Autodesk Fusion 360 part; units mm, degrees
(part 2 of 2)
sketch "Sketch2 (2)" plane through (0, 0, 0) normal (-1, 0, 0) x (0, -1, 0) in component "left"
  line L0 (-22.5, 130) -> (-22.5, 127)
  line L1 (-22.5, 127) -> (-32.1429, 127)
  line L2 (-32.1429, 127) -> (-32.1429, 130)
  line L3 (-32.1429, 130) -> (-42.8571, 130)
  line L4 (-42.8571, 130) -> (-42.8571, 127)
  line L5 (-42.8571, 127) -> (-52.5, 127)
  line L6 (-52.5, 127) -> (-52.5, 130)
  line L7 (-52.5, 130) -> (-52.5, 200)
  line L8 (-52.5, 200) -> (-72, 200)
  line L9 (-72, 200) -> (-72, 177.7778)
  line L10 (-72, 177.7778) -> (-75, 177.7778)
  line L11 (-75, 177.7778) -> (-75, 155.5556)
  line L12 (-75, 155.5556) -> (-72, 155.5556)
  line L13 (-72, 155.5556) -> (-72, 133.3333)
  line L14 (-72, 133.3333) -> (-75, 133.3333)
  line L15 (-75, 133.3333) -> (-75, 111.1111)
  line L16 (-75, 111.1111) -> (-72, 111.1111)
  line L17 (-72, 111.1111) -> (-72, 88.8889)
  line L18 (-72, 88.8889) -> (-75, 88.8889)
  line L19 (-75, 88.8889) -> (-75, 66.6667)
  line L20 (-75, 66.6667) -> (-72, 66.6667)
  line L21 (-72, 66.6667) -> (-72, 44.4444)
  line L22 (-72, 44.4444) -> (-75, 44.4444)
  line L23 (-75, 44.4444) -> (-75, 22.2222)
  line L24 (-75, 22.2222) -> (-72, 22.2222)
  line L25 (-72, 22.2222) -> (-72, 3)
  line L26 (-72, 3) -> (-64.2857, 3)
  line L27 (-64.2857, 3) -> (-64.2857, 0)
  line L28 (-64.2857, 0) -> (-53.5714, 0)
  line L29 (-53.5714, 0) -> (-53.5714, 3)
  line L30 (-53.5714, 3) -> (-42.8571, 3)
  line L31 (-42.8571, 3) -> (-42.8571, 0)
  line L32 (-42.8571, 0) -> (-32.1429, 0)
  line L33 (-32.1429, 0) -> (-32.1429, 3)
  line L34 (-32.1429, 3) -> (-21.4286, 3)
  line L35 (-21.4286, 3) -> (-21.4286, 0)
  line L36 (-21.4286, 0) -> (-10.7143, 0)
  line L37 (-10.7143, 0) -> (-10.7143, 3)
  line L38 (-10.7143, 3) -> (-3, 3)
  line L39 (-3, 3) -> (-3, 22.2222)
  line L40 (-3, 22.2222) -> (0, 22.2222)
  line L41 (0, 22.2222) -> (0, 44.4444)
  line L42 (0, 44.4444) -> (-3, 44.4444)
  line L43 (-3, 44.4444) -> (-3, 66.6667)
  line L44 (-3, 66.6667) -> (0, 66.6667)
  line L45 (0, 66.6667) -> (0, 88.8889)
  line L46 (0, 88.8889) -> (-3, 88.8889)
  line L47 (-3, 88.8889) -> (-3, 111.1111)
  line L48 (-3, 111.1111) -> (0, 111.1111)
  line L49 (0, 111.1111) -> (0, 133.3333)
  line L50 (0, 133.3333) -> (-3, 133.3333)
  line L51 (-3, 133.3333) -> (-3, 155.5556)
  line L52 (-3, 155.5556) -> (0, 155.5556)
  line L53 (0, 155.5556) -> (0, 177.7778)
  line L54 (0, 177.7778) -> (-3, 177.7778)
  line L55 (-3, 177.7778) -> (-3, 200)
  line L56 (-3, 200) -> (-22.5, 200)
  line L57 (-22.5, 200) -> (-22.5, 130)
  line L58 (-52.5, 200) -> (-22.5, 200)
  line L59 (-22.5, 200) -> (-22.5, 156)
  line L60 (-22.5, 156) -> (-52.5, 156)
  line L61 (-52.5, 156) -> (-52.5, 200)
  dimension "d161" = 26
  constraint horizontal L58
  constraint vertical L59
  constraint horizontal L60
  constraint vertical L61
  constraint coincident L57 L59.end
  constraint coincident L7.end L8.start
  measures "d161" distance of L3 L60
extrude "Extrude4'''" add sketch "Sketch2 (2)" against normal blind 3 contours L7 L57 L58 L59 L60 L61 bodies 5 in component "left"
combine "Combine6" operation cut target body 4 tool bodies 8 keep tools in component "right"
sketch "Sketch3 (2)" plane through (0, 0, 0) normal (-1, 0, 0) x (0, -1, 0) in component "left"
  line L0 (-22.5, 156) -> (-22.5, 130)
  line L1 (-22.5, 130) -> (-22.5, 127)
  line L2 (-22.5, 127) -> (-32.1429, 127)
  line L3 (-32.1429, 127) -> (-32.1429, 130)
  line L4 (-32.1429, 130) -> (-42.8571, 130)
  line L5 (-42.8571, 130) -> (-42.8571, 127)
  line L6 (-42.8571, 127) -> (-52.5, 127)
  line L7 (-52.5, 127) -> (-52.5, 130)
  line L8 (-52.5, 130) -> (-52.5, 156)
  line L9 (-52.5, 156) -> (-22.5, 156)
  line L10 (-3, 200) -> (-72, 200)
  line L11 (-72, 200) -> (-72, 177.7778)
  line L12 (-72, 177.7778) -> (-75, 177.7778)
  line L13 (-75, 177.7778) -> (-75, 155.5556)
  line L14 (-75, 155.5556) -> (-72, 155.5556)
  line L15 (-72, 155.5556) -> (-72, 133.3333)
  line L16 (-72, 133.3333) -> (-75, 133.3333)
  line L17 (-75, 133.3333) -> (-75, 111.1111)
  line L18 (-75, 111.1111) -> (-72, 111.1111)
  line L19 (-72, 111.1111) -> (-72, 88.8889)
  line L20 (-72, 88.8889) -> (-75, 88.8889)
  line L21 (-75, 88.8889) -> (-75, 66.6667)
  line L22 (-75, 66.6667) -> (-72, 66.6667)
  line L23 (-72, 66.6667) -> (-72, 44.4444)
  line L24 (-72, 44.4444) -> (-75, 44.4444)
  line L25 (-75, 44.4444) -> (-75, 22.2222)
  line L26 (-75, 22.2222) -> (-72, 22.2222)
  line L27 (-72, 22.2222) -> (-72, 3)
  line L28 (-72, 3) -> (-64.2857, 3)
  line L29 (-64.2857, 3) -> (-64.2857, 0)
  line L30 (-64.2857, 0) -> (-53.5714, 0)
  line L31 (-53.5714, 0) -> (-53.5714, 3)
  line L32 (-53.5714, 3) -> (-42.8571, 3)
  line L33 (-42.8571, 3) -> (-42.8571, 0)
  line L34 (-42.8571, 0) -> (-32.1429, 0)
  line L35 (-32.1429, 0) -> (-32.1429, 3)
  line L36 (-32.1429, 3) -> (-21.4286, 3)
  line L37 (-21.4286, 3) -> (-21.4286, 0)
  line L38 (-21.4286, 0) -> (-10.7143, 0)
  line L39 (-10.7143, 0) -> (-10.7143, 3)
  line L40 (-10.7143, 3) -> (-3, 3)
  line L41 (-3, 3) -> (-3, 22.2222)
  line L42 (-3, 22.2222) -> (0, 22.2222)
  line L43 (0, 22.2222) -> (0, 44.4444)
  line L44 (0, 44.4444) -> (-3, 44.4444)
  line L45 (-3, 44.4444) -> (-3, 66.6667)
  line L46 (-3, 66.6667) -> (0, 66.6667)
  line L47 (0, 66.6667) -> (0, 88.8889)
  line L48 (0, 88.8889) -> (-3, 88.8889)
  line L49 (-3, 88.8889) -> (-3, 111.1111)
  line L50 (-3, 111.1111) -> (0, 111.1111)
  line L51 (0, 111.1111) -> (0, 133.3333)
  line L52 (0, 133.3333) -> (-3, 133.3333)
  line L53 (-3, 133.3333) -> (-3, 155.5556)
  line L54 (-3, 155.5556) -> (0, 155.5556)
  line L55 (0, 155.5556) -> (0, 177.7778)
  line L56 (0, 177.7778) -> (-3, 177.7778)
  line L57 (-3, 177.7778) -> (-3, 200)
  circle A0 centre (-60, 117) radius 2.5
  dimension "d164" = 10
  dimension "d165" = 5
  dimension "d166" = 15
  measures "d164" distance of L6 A0.centre
  measures "d165" diameter of A0
  measures "d166" distance of L17 A0.centre
extrude "Extrude5'''" cut sketch "Sketch3 (2)" against normal blind 3 contours A0 bodies 5 in component "left"
sketch "Sketch7" plane through (75, 0, 0) normal (1, 0, 0) x (0, 1, 0) in component "right"
  line L0 (72, 78) -> (72, 66.6667)
  line L1 (72, 66.6667) -> (75, 66.6667)
  line L2 (75, 66.6667) -> (75, 88.8889)
  line L3 (75, 88.8889) -> (72, 88.8889)
  line L4 (72, 88.8889) -> (72, 111.1111)
  line L5 (72, 111.1111) -> (75, 111.1111)
  line L6 (75, 111.1111) -> (75, 133.3333)
  line L7 (75, 133.3333) -> (72, 133.3333)
  line L8 (72, 133.3333) -> (72, 155.5556)
  line L9 (72, 155.5556) -> (75, 155.5556)
  line L10 (75, 155.5556) -> (75, 177.7778)
  line L11 (75, 177.7778) -> (72, 177.7778)
  line L12 (72, 177.7778) -> (72, 200)
  line L13 (72, 200) -> (3, 200)
  line L14 (3, 200) -> (3, 177.7778)
  line L15 (3, 177.7778) -> (0, 177.7778)
  line L16 (0, 177.7778) -> (0, 155.5556)
  line L17 (0, 155.5556) -> (3, 155.5556)
  line L18 (3, 155.5556) -> (3, 133.3333)
  line L19 (3, 133.3333) -> (0, 133.3333)
  line L20 (0, 133.3333) -> (0, 111.1111)
  line L21 (0, 111.1111) -> (3, 111.1111)
  line L22 (3, 111.1111) -> (3, 88.8889)
  line L23 (3, 88.8889) -> (0, 88.8889)
  line L24 (0, 88.8889) -> (0, 66.6667)
  line L25 (0, 66.6667) -> (3, 66.6667)
  line L26 (3, 66.6667) -> (3, 44.4444)
  line L27 (3, 44.4444) -> (0, 44.4444)
  line L28 (0, 44.4444) -> (0, 22.2222)
  line L29 (0, 22.2222) -> (3, 22.2222)
  line L30 (3, 22.2222) -> (3, 3)
  line L31 (3, 3) -> (10.7143, 3)
  line L32 (10.7143, 3) -> (10.7143, 0)
  line L33 (10.7143, 0) -> (21.4286, 0)
  line L34 (21.4286, 0) -> (21.4286, 3)
  line L35 (21.4286, 3) -> (32.1429, 3)
  line L36 (32.1429, 3) -> (32.1429, 0)
  line L37 (32.1429, 0) -> (42.8571, 0)
  line L38 (42.8571, 0) -> (42.8571, 3)
  line L39 (42.8571, 3) -> (53.5714, 3)
  line L40 (53.5714, 3) -> (53.5714, 0)
  line L41 (53.5714, 0) -> (64.2857, 0)
  line L42 (64.2857, 0) -> (64.2857, 3)
  line L43 (64.2857, 3) -> (69, 3)
  line L44 (69, 3) -> (69, 78)
  line L45 (69, 78) -> (72, 78)
  circle A0 centre (60, 117) radius 2.5
  line L46 (52.5, 127) -> (42.8571, 127)
  line L47 (75, 0) -> (75, 200)
  dimension "d171" = 5
  dimension "d190" = 10
  dimension "d191" = 15
  measures "d171" diameter of A0
  measures "d190" distance of A0.centre L46
  measures "d191" distance of A0.centre L47
extrude "Extrude8" cut sketch "Sketch7" against normal blind 8 contours A0 bodies 4 in component "right"
sketch "Sketch3 (3)" plane through (0, 0, 0) normal (0, -1, 0) x (1, 0, 0) in component "front"
  line L0 (52.5, 156) -> (52.5, 130)
  line L1 (52.5, 130) -> (50, 130)
  line L2 (50, 130) -> (50, 127)
  line L3 (50, 127) -> (41.6667, 127)
  line L4 (41.6667, 127) -> (41.6667, 130)
  line L5 (41.6667, 130) -> (33.3333, 130)
  line L6 (33.3333, 130) -> (33.3333, 127)
  line L7 (33.3333, 127) -> (25, 127)
  line L8 (25, 127) -> (25, 130)
  line L9 (25, 130) -> (22.5, 130)
  line L10 (22.5, 130) -> (22.5, 156)
  line L11 (22.5, 156) -> (52.5, 156)
  line L12 (75, 200) -> (0, 200)
  line L13 (0, 200) -> (0, 177.7778)
  line L14 (0, 177.7778) -> (3, 177.7778)
  line L15 (3, 177.7778) -> (3, 155.5556)
  line L16 (3, 155.5556) -> (0, 155.5556)
  line L17 (0, 155.5556) -> (0, 133.3333)
  line L18 (0, 133.3333) -> (3, 133.3333)
  line L19 (3, 133.3333) -> (3, 111.1111)
  line L20 (3, 111.1111) -> (0, 111.1111)
  line L21 (0, 111.1111) -> (0, 88.8889)
  line L22 (0, 88.8889) -> (3, 88.8889)
  line L23 (3, 88.8889) -> (3, 66.6667)
  line L24 (3, 66.6667) -> (0, 66.6667)
  line L25 (0, 66.6667) -> (0, 44.4444)
  line L26 (0, 44.4444) -> (3, 44.4444)
  line L27 (3, 44.4444) -> (3, 22.2222)
  line L28 (3, 22.2222) -> (0, 22.2222)
  line L29 (0, 22.2222) -> (0, 3)
  line L30 (0, 3) -> (8.3333, 3)
  line L31 (8.3333, 3) -> (8.3333, 0)
  line L32 (8.3333, 0) -> (16.6667, 0)
  line L33 (16.6667, 0) -> (16.6667, 3)
  line L34 (16.6667, 3) -> (25, 3)
  line L35 (25, 3) -> (25, 0)
  line L36 (25, 0) -> (33.3333, 0)
  line L37 (33.3333, 0) -> (33.3333, 3)
  line L38 (33.3333, 3) -> (41.6667, 3)
  line L39 (41.6667, 3) -> (41.6667, 0)
  line L40 (41.6667, 0) -> (50, 0)
  line L41 (50, 0) -> (50, 3)
  line L42 (50, 3) -> (58.3333, 3)
  line L43 (58.3333, 3) -> (58.3333, 0)
  line L44 (58.3333, 0) -> (66.6667, 0)
  line L45 (66.6667, 0) -> (66.6667, 3)
  line L46 (66.6667, 3) -> (75, 3)
  line L47 (75, 3) -> (75, 22.2222)
  line L48 (75, 22.2222) -> (72, 22.2222)
  line L49 (72, 22.2222) -> (72, 44.4444)
  line L50 (72, 44.4444) -> (75, 44.4444)
  line L51 (75, 44.4444) -> (75, 66.6667)
  line L52 (75, 66.6667) -> (72, 66.6667)
  line L53 (72, 66.6667) -> (72, 88.8889)
  line L54 (72, 88.8889) -> (75, 88.8889)
  line L55 (75, 88.8889) -> (75, 111.1111)
  line L56 (75, 111.1111) -> (72, 111.1111)
  line L57 (72, 111.1111) -> (72, 133.3333)
  line L58 (72, 133.3333) -> (75, 133.3333)
  line L59 (75, 133.3333) -> (75, 155.5556)
  line L60 (75, 155.5556) -> (72, 155.5556)
  line L61 (72, 155.5556) -> (72, 177.7778)
  line L62 (72, 177.7778) -> (75, 177.7778)
  line L63 (75, 177.7778) -> (75, 200)
  circle A0 centre (18, 117) radius 2.5
  dimension "d174" = 10
  dimension "d175" = 15
  dimension "d176" = 5
  measures "d174" distance of L7 A0.centre
  measures "d175" distance of L19 A0.centre
  measures "d176" diameter of A0
extrude "Extrude5''''" cut sketch "Sketch3 (3)" against normal blind 3 contours A0 bodies 3 in component "front"
sketch "Sketch6 (2)" plane through (0, 72, 0) normal (0, -1, 0) x (1, 0, 0) in component "back"
  line L0 (13, 8) -> (13, 78)
  line L1 (13, 78) -> (62, 78)
  line L2 (62, 78) -> (62, 8)
  line L3 (62, 8) -> (13, 8)
  line L4 (0, 3) -> (8.3333, 3)
  line L5 (8.3333, 3) -> (8.3333, 0)
  line L6 (8.3333, 0) -> (16.6667, 0)
  line L7 (16.6667, 0) -> (16.6667, 3)
  line L8 (16.6667, 3) -> (25, 3)
  line L9 (25, 3) -> (25, 0)
  line L10 (25, 0) -> (33.3333, 0)
  line L11 (33.3333, 0) -> (33.3333, 3)
  line L12 (33.3333, 3) -> (41.6667, 3)
  line L13 (41.6667, 3) -> (41.6667, 0)
  line L14 (41.6667, 0) -> (50, 0)
  line L15 (50, 0) -> (50, 3)
  line L16 (50, 3) -> (58.3333, 3)
  line L17 (58.3333, 3) -> (58.3333, 0)
  line L18 (58.3333, 0) -> (66.6667, 0)
  line L19 (66.6667, 0) -> (66.6667, 3)
  line L20 (66.6667, 3) -> (75, 3)
  line L21 (75, 3) -> (75, 22.2222)
  line L22 (75, 22.2222) -> (75, 44.4444)
  line L23 (75, 44.4444) -> (75, 66.6667)
  line L24 (75, 66.6667) -> (72, 66.6667)
  line L25 (72, 66.6667) -> (72, 88.8889)
  line L26 (72, 88.8889) -> (75, 88.8889)
  line L27 (75, 88.8889) -> (75, 111.1111)
  line L28 (75, 111.1111) -> (72, 111.1111)
  line L29 (72, 111.1111) -> (72, 133.3333)
  line L30 (72, 133.3333) -> (75, 133.3333)
  line L31 (75, 133.3333) -> (75, 155.5556)
  line L32 (75, 155.5556) -> (72, 155.5556)
  line L33 (72, 155.5556) -> (72, 177.7778)
  line L34 (72, 177.7778) -> (75, 177.7778)
  line L35 (75, 177.7778) -> (75, 200)
  line L36 (75, 200) -> (0, 200)
  line L37 (0, 200) -> (0, 177.7778)
  line L38 (0, 177.7778) -> (3, 177.7778)
  line L39 (3, 177.7778) -> (3, 155.5556)
  line L40 (3, 155.5556) -> (0, 155.5556)
  line L41 (0, 155.5556) -> (0, 133.3333)
  line L42 (0, 133.3333) -> (3, 133.3333)
  line L43 (3, 133.3333) -> (3, 111.1111)
  line L44 (3, 111.1111) -> (0, 111.1111)
  line L45 (0, 111.1111) -> (0, 88.8889)
  line L46 (0, 88.8889) -> (3, 88.8889)
  line L47 (3, 88.8889) -> (3, 66.6667)
  line L48 (3, 66.6667) -> (0, 66.6667)
  line L49 (0, 66.6667) -> (0, 44.4444)
  line L50 (0, 44.4444) -> (3, 44.4444)
  line L51 (3, 44.4444) -> (3, 22.2222)
  line L52 (3, 22.2222) -> (0, 22.2222)
  line L53 (0, 22.2222) -> (0, 3)
  circle A0 centre (37.5, 117) radius 2.5
  line L54 (3, 127) -> (72, 127)
  line L55 (37.5, 117) -> (37.5, 127)
  dimension "d183" = 5
  dimension "d186" = 10
  constraint coincident A0.centre L55.start
  constraint coincident L54 L55.end
  constraint perpendicular L54 L55
  constraint midpoint L54 L55.end
  measures "d183" diameter of A0
  measures "d186" distance of A0.centre L55.end
extrude "Extrude7'" cut sketch "Sketch6 (2)" against normal blind 6 contours A0 bodies 2 in component "back"
extrude "Extrude9" cut sketch "spout_cut" against normal blind 10 contours L30 L48 L49 L50 L51 bodies 4 in component "right"
sketch "Sketch8" plane through (75, 0, 0) normal (1, 0, 0) x (0, 1, 0) in component "right"
  line L0 (52.5, 156) -> (22.5, 156)
  line L1 (22.5, 156) -> (22.5, 200)
  line L2 (22.5, 200) -> (52.5, 200)
  line L3 (52.5, 200) -> (52.5, 156)
  line L4 (22.5, 156) -> (52.5, 156)
  line L5 (52.5, 200) -> (52.5, 130)
  point P0 (22.5, 200)
  constraint horizontal L0
  constraint vertical L1
  constraint horizontal L2
  constraint vertical L3
  constraint coincident P0 L1.end
  constraint coincident L0.start L4
  constraint coincident L2.end L5
extrude "Extrude10" add sketch "Sketch8" against normal blind 3 bodies 4 in component "right"
combine "Combine7" operation cut target body 4 tool bodies 6 keep tools in component "right"
sketch "Sketch1 (5)" plane through (0, 0, 200) normal (0, 0, 1) x (-1, 0, 0) in component "cover"
  line L0 (-75, -75) -> (0, -75)
  line L1 (0, -75) -> (0, -72)
  line L2 (0, -72) -> (-75, -72)
  line L3 (-75, -72) -> (-75, -75)
  line L4 (-75, -75) -> (0, -75)
  line L5 (0, -75) -> (0, 0)
  line L6 (0, 0) -> (-75, 0)
  line L7 (-75, 0) -> (-75, -75)
  line L8 (5, 5) -> (-80, 5)
  line L9 (-80, 5) -> (-80, -80)
  line L10 (-80, -80) -> (5, -80)
  line L11 (5, -80) -> (5, 5)
  line L12 (0, -64.2857) -> (-3, -64.2857)
  line L13 (-3, -64.2857) -> (-3, -53.5714)
  line L14 (-3, -53.5714) -> (0, -53.5714)
  line L15 (0, -53.5714) -> (0, -64.2857)
  line L16 (0, -64.2857) -> (-3, -64.2857)
  line L17 (-3, -53.5714) -> (0, -53.5714)
  line L18 (-3, -42.8571) -> (0, -42.8571)
  line L19 (0, -42.8571) -> (0, -32.1429)
  line L20 (0, -32.1429) -> (-3, -32.1429)
  line L21 (-3, -32.1429) -> (-3, -42.8571)
  line L22 (-3, -21.4286) -> (0, -21.4286)
  line L23 (0, -21.4286) -> (0, -10.7143)
  line L24 (0, -10.7143) -> (-3, -10.7143)
  line L25 (-3, -10.7143) -> (-3, -21.4286)
  line L26 (0, -21.4286) -> (-3, -21.4286)
  line L27 (-3, -32.1429) -> (0, -32.1429)
  line L28 (-16.6667, -75) -> (-8.3333, -75)
  line L29 (-8.3333, -75) -> (-8.3333, -72)
  line L30 (-8.3333, -72) -> (-16.6667, -72)
  line L31 (-16.6667, -72) -> (-16.6667, -75)
  line L32 (-33.3333, -75) -> (-25, -75)
  line L33 (-25, -75) -> (-25, -72)
  line L34 (-25, -72) -> (-33.3333, -72)
  line L35 (-33.3333, -72) -> (-33.3333, -75)
  line L36 (-50, -75) -> (-41.6667, -75)
  line L37 (-41.6667, -75) -> (-41.6667, -72)
  line L38 (-41.6667, -72) -> (-50, -72)
  line L39 (-50, -72) -> (-50, -75)
  line L40 (-66.6667, -75) -> (-58.3333, -75)
  line L41 (-58.3333, -75) -> (-58.3333, -72)
  line L42 (-58.3333, -72) -> (-66.6667, -72)
  line L43 (-66.6667, -72) -> (-66.6667, -75)
  line L44 (-8.3333, -72) -> (-8.3333, -75)
  line L45 (-16.6667, -75) -> (-16.6667, -72)
  line L46 (-25, -72) -> (-25, -75)
  line L47 (-33.3333, -75) -> (-33.3333, -72)
  line L48 (-41.6667, -72) -> (-41.6667, -75)
  line L49 (-58.3333, -72) -> (-58.3333, -75)
  line L50 (-66.6667, -75) -> (-66.6667, -72)
  line L51 (5, -37.5) -> (-80, -37.5) construction
  line L52 (-37.5, -80) -> (-37.5, 5) construction
  line L53 (-72, -42.8571) -> (-75, -42.8571)
  line L54 (-75, -21.4286) -> (-75, -10.7143)
  line L55 (-72, -64.2857) -> (-72, -53.5714)
  line L56 (-75, -64.2857) -> (-72, -64.2857)
  line L57 (-72, -32.1429) -> (-72, -42.8571)
  line L58 (-75, -42.8571) -> (-75, -32.1429)
  line L59 (-72, -53.5714) -> (-75, -53.5714)
  line L60 (-75, -64.2857) -> (-72, -64.2857)
  line L61 (-72, -32.1429) -> (-75, -32.1429)
  line L62 (-75, -32.1429) -> (-72, -32.1429)
  line L63 (-75, -10.7143) -> (-72, -10.7143)
  line L64 (-72, -53.5714) -> (-75, -53.5714)
  line L65 (-75, -75) -> (-75, 0)
  line L66 (-75, -53.5714) -> (-75, -64.2857)
  line L67 (-80, -37.5) -> (5, -37.5) construction
  line L68 (-72, -10.7143) -> (-72, -21.4286)
  line L69 (-72, -21.4286) -> (-75, -21.4286)
  line L70 (-75, -21.4286) -> (-72, -21.4286)
  line L71 (-16.6667, -3) -> (-16.6667, 0)
  line L72 (-16.6667, 0) -> (-8.3333, 0)
  line L73 (-33.3333, -3) -> (-33.3333, 0)
  line L74 (-50, 0) -> (-41.6667, 0)
  line L75 (-8.3333, -3) -> (-16.6667, -3)
  line L76 (-41.6667, -3) -> (-50, -3)
  line L77 (-58.3333, 0) -> (-58.3333, -3)
  line L78 (-41.6667, -3) -> (-41.6667, 0)
  line L79 (-58.3333, -3) -> (-66.6667, -3)
  line L80 (-33.3333, 0) -> (-25, 0)
  line L81 (-25, 0) -> (-25, -3)
  line L82 (-8.3333, 0) -> (-8.3333, -3)
  line L83 (-8.3333, -3) -> (-8.3333, 0)
  line L84 (-66.6667, -3) -> (-66.6667, 0)
  line L85 (-66.6667, 0) -> (-58.3333, 0)
  line L86 (-25, -3) -> (-25, 0)
  line L87 (-66.6667, 0) -> (-66.6667, -3)
  line L88 (-25, -3) -> (-33.3333, -3)
  line L89 (-58.3333, -3) -> (-58.3333, 0)
  line L90 (-41.6667, 0) -> (-41.6667, -3)
  line L91 (-16.6667, 0) -> (-16.6667, -3)
  line L92 (-50, -3) -> (-50, 0)
  line L93 (-33.3333, 0) -> (-33.3333, -3)
  point P0 (-3, -42.8571)
  point P1 (-3, -10.7143)
  point P2 (-50, -72)
  point P3 (-72, -42.8571)
  point P4 (-72, -10.7143)
  point P5 (-50, -3)
  dimension "d199" = 5
  constraint horizontal L4
  constraint vertical L5
  constraint horizontal L6
  constraint vertical L7
  constraint coincident L5.end L6.start
  constraint coincident L0.start L3.end
  constraint horizontal L12
  constraint vertical L13
  constraint horizontal L14
  constraint vertical L15
  constraint coincident L5 L12.start
  constraint coincident L12.end L16
  constraint coincident L13.end L17
  constraint horizontal L18
  constraint vertical L19
  constraint horizontal L20
  constraint vertical L21
  constraint horizontal L22
  constraint vertical L23
  constraint horizontal L24
  constraint vertical L25
  constraint coincident L5 L23.end
  constraint coincident L22.start L26
  constraint coincident L20.end L27
  constraint coincident P0 L18.start
  constraint coincident L13 L12.end
  constraint coincident P1 L24.end
  constraint horizontal L28
  constraint vertical L29
  constraint horizontal L30
  constraint vertical L31
  constraint coincident L2 L29.end
  constraint coincident L4 L28.start
  constraint horizontal L32
  constraint vertical L33
  constraint horizontal L34
  constraint vertical L35
  constraint coincident L2 L33.end
  constraint coincident L4 L32.start
  constraint horizontal L36
  constraint vertical L37
  constraint horizontal L38
  constraint vertical L39
  constraint coincident L2 L37.end
  constraint coincident L4 L36.start
  constraint horizontal L40
  constraint vertical L41
  constraint horizontal L42
  constraint vertical L43
  constraint coincident L2 L41.end
  constraint coincident L4 L40.start
  constraint coincident L29.end L44
  constraint coincident L30.end L45
  constraint coincident L33.end L46
  constraint coincident L34.end L47
  constraint coincident L37.end L48
  constraint coincident L39 P2
  constraint coincident L41.end L49
  constraint coincident L42.end L50
  constraint midpoint L11 L51.start
  constraint midpoint L9 L51.end
  constraint midpoint L10 L52.start
  constraint midpoint L8 L52.end
  constraint symmetric L0.end L52 L0.start
  constraint symmetric L5.end L52 L6.end
  constraint symmetric L12.start L52 L56.start
  constraint symmetric L12.end L52 L55.start
  constraint symmetric L13.end L52 L55.end
  constraint symmetric L14.end L52 L59.end
  constraint symmetric P0 L52 P3
  constraint symmetric L18.end L52 L53.end
  constraint symmetric L19.end L52 L58.end
  constraint symmetric L20.end L52 L57.start
  constraint symmetric L22.start L52 L68.end
  constraint symmetric L22.end L52 L54.start
  constraint symmetric L23.end L52 L54.end
  constraint symmetric P1 L52 P4
  constraint symmetric L51.start L52 L51.end
  constraint symmetric L51.end L52 L51.start
  constraint symmetric L28.start L51 L71.end
  constraint symmetric L28.end L51 L72.end
  constraint symmetric L29.end L51 L75.start
  constraint symmetric L30.end L51 L71.start
  constraint symmetric L32.start L51 L73.end
  constraint symmetric L32.end L51 L80.end
  constraint symmetric L33.end L51 L81.end
  constraint symmetric L34.end L51 L73.start
  constraint symmetric L36.start L51 L74.start
  constraint symmetric L36.end L51 L74.end
  constraint symmetric L37.end L51 L76.start
  constraint symmetric P2 L51 P5
  constraint symmetric L40.start L51 L84.end
  constraint symmetric L40.end L51 L77.start
  constraint symmetric L41.end L51 L77.end
  constraint symmetric L42.end L51 L79.end
extrude "Extrude1'''''''" add sketch "Sketch1 (5)" against normal blind 3 separate body contours L0 L2 L3 L4 L7 L43 L50 L65 | L2 L5 L6 L7 L12 L13 L14 L16 L17 L18 L20 L21 L22 L24 L25 L26 L27 L30 L34 L38 L42 L53 L55 L56 L57 L59 L60 L61 L62 L63 L64 L65 L68 L69 L70 L71 L73 L75 L76 L77 L78 L79 L81 L82 L83 L84 L86 L87 L88 L89 L90 L91 L92 L93 | L0 L2 L4 L39 L41 L49 | L0 L2 L4 L35 L37 L47 L48 | L0 L2 L4 L31 L33 L45 L46 | L0 L1 L2 L4 L5 L29 L44 | L8 L9 L10 L11 makes body 9 in component "cover"
combine "Combine5'" operation cut target body 3 tool bodies 9 keep tools in component "front"
combine "Combine9" operation cut target body 4 tool bodies 9 keep tools in component "right"
combine "Combine5''" operation cut target body 2 tool bodies 9 keep tools in component "back"
combine "Combine4'" operation cut target body 5 tool bodies 9 keep tools in component "left"
sketch "Sketch7 (2)" plane through (0, 75, 0) normal (0, 1, 0) x (-1, 0, 0) in component "back"
  line L0 (-13, 78) -> (-13, 8)
  line L1 (-13, 8) -> (-62, 8)
  line L2 (-62, 8) -> (-62, 78)
  line L3 (-62, 78) -> (-13, 78)
  circle A0 centre (-37.5, 117) radius 2.5
  line L4 (0, 197) -> (-8.3333, 197)
  line L5 (-8.3333, 197) -> (-8.3333, 200)
  line L6 (-8.3333, 200) -> (-16.6667, 200)
  line L7 (-16.6667, 200) -> (-16.6667, 197)
  line L8 (-16.6667, 197) -> (-25, 197)
  line L9 (-25, 197) -> (-25, 200)
  line L10 (-25, 200) -> (-33.3333, 200)
  line L11 (-33.3333, 200) -> (-33.3333, 197)
  line L12 (-33.3333, 197) -> (-41.6667, 197)
  line L13 (-41.6667, 197) -> (-41.6667, 200)
  line L14 (-41.6667, 200) -> (-50, 200)
  line L15 (-50, 200) -> (-50, 197)
  line L16 (-50, 197) -> (-58.3333, 197)
  line L17 (-58.3333, 197) -> (-58.3333, 200)
  line L18 (-58.3333, 200) -> (-66.6667, 200)
  line L19 (-66.6667, 200) -> (-66.6667, 197)
  line L20 (-66.6667, 197) -> (-75, 197)
  line L21 (-75, 197) -> (-75, 177.7778)
  line L22 (-75, 177.7778) -> (-72, 177.7778)
  line L23 (-72, 177.7778) -> (-72, 155.5556)
  line L24 (-72, 155.5556) -> (-75, 155.5556)
  line L25 (-75, 155.5556) -> (-75, 133.3333)
  line L26 (-75, 133.3333) -> (-72, 133.3333)
  line L27 (-72, 133.3333) -> (-72, 111.1111)
  line L28 (-72, 111.1111) -> (-75, 111.1111)
  line L29 (-75, 111.1111) -> (-75, 88.8889)
  line L30 (-75, 88.8889) -> (-72, 88.8889)
  line L31 (-72, 88.8889) -> (-72, 66.6667)
  line L32 (-72, 66.6667) -> (-75, 66.6667)
  line L33 (-75, 66.6667) -> (-75, 44.4444)
  line L34 (-75, 44.4444) -> (-75, 22.2222)
  line L35 (-75, 22.2222) -> (-75, 3)
  line L36 (-75, 3) -> (-66.6667, 3)
  line L37 (-66.6667, 3) -> (-66.6667, 0)
  line L38 (-66.6667, 0) -> (-58.3333, 0)
  line L39 (-58.3333, 0) -> (-58.3333, 3)
  line L40 (-58.3333, 3) -> (-50, 3)
  line L41 (-50, 3) -> (-50, 0)
  line L42 (-50, 0) -> (-41.6667, 0)
  line L43 (-41.6667, 0) -> (-41.6667, 3)
  line L44 (-41.6667, 3) -> (-33.3333, 3)
  line L45 (-33.3333, 3) -> (-33.3333, 0)
  line L46 (-33.3333, 0) -> (-25, 0)
  line L47 (-25, 0) -> (-25, 3)
  line L48 (-25, 3) -> (-16.6667, 3)
  line L49 (-16.6667, 3) -> (-16.6667, 0)
  line L50 (-16.6667, 0) -> (-8.3333, 0)
  line L51 (-8.3333, 0) -> (-8.3333, 3)
  line L52 (-8.3333, 3) -> (0, 3)
  line L53 (0, 3) -> (0, 22.2222)
  line L54 (0, 22.2222) -> (-3, 22.2222)
  line L55 (-3, 22.2222) -> (-3, 44.4444)
  line L56 (-3, 44.4444) -> (0, 44.4444)
  line L57 (0, 44.4444) -> (0, 66.6667)
  line L58 (0, 66.6667) -> (-3, 66.6667)
  line L59 (-3, 66.6667) -> (-3, 88.8889)
  line L60 (-3, 88.8889) -> (0, 88.8889)
  line L61 (0, 88.8889) -> (0, 111.1111)
  line L62 (0, 111.1111) -> (-3, 111.1111)
  line L63 (-3, 111.1111) -> (-3, 133.3333)
  line L64 (-3, 133.3333) -> (0, 133.3333)
  line L65 (0, 133.3333) -> (0, 155.5556)
  line L66 (0, 155.5556) -> (-3, 155.5556)
  line L67 (-3, 155.5556) -> (-3, 177.7778)
  line L68 (-3, 177.7778) -> (0, 177.7778)
  line L69 (0, 177.7778) -> (0, 197)
  circle A1 centre (-37.5, 182) radius 5
  line L70 (-37.5, 197) -> (-37.5, 167)
  dimension "d202" = 10
  dimension "d203" = 15
  constraint midpoint L12 L70.start
  constraint perpendicular L12 L70
  constraint coincident A1.centre L70
  measures "d202" diameter of A1
  measures "d203" distance of L12 A1.centre
extrude "Extrude8'" cut sketch "Sketch7 (2)" against normal blind 6 contours A1 L70 | A1 L70 bodies 2 in component "back"
component "base" placed x (1, 0, 0) y (0, 1, 0) z (0, 0, 1) at (0, 0, 0)
component "back" placed x (1, 0, 0) y (0, 1, 0) z (0, 0, 1) at (0, 0, 0)
component "front" placed x (1, 0, 0) y (0, 1, 0) z (0, 0, 1) at (0, 0, 0)
component "right" placed x (1, 0, 0) y (0, 1, 0) z (0, 0, 1) at (0, 0, 0)
component "left" placed x (1, 0, 0) y (0, 1, 0) z (0, 0, 1) at (0, 0, 0)
component "mid panel" placed x (1, 0, 0) y (0, 1, 0) z (0, 0, 1) at (0, 0, 0)
component "slider guide" placed x (1, 0, 0) y (0, 1, 0) z (0, 0, 1) at (0, 0, 0)
component "slide door" placed x (1, 0, 0) y (0, 1, 0) z (0, 0, 1) at (0, 0, 0)
component "cover" placed x (1, 0, 0) y (0, 1, 0) z (0, 0, 1) at (0, 0, 0)
equation "length = 75 mm" comment "exterior"
equation "width = 75 mm" comment "exterior"
equation "height = 200 mm" comment "exterior"
equation "thick = 3 mm" comment "material thickness"
equation "Ltab = 4" comment "No. tab"
equation "Wtab = 3" comment "No. tab"
equation "Htab = 4" comment "No. tab"
equation "WtabWidth = width / ( ( Wtab * 2 ) + 1 )" comment "tab size"
equation "LtabWidth = length / ( ( Ltab * 2 ) + 1 )" comment "tab size"
equation "HtabWidth = height / ( ( Htab * 2 ) + 1 )" comment "tab size"
equation "baseoffset = 5 mm" comment "Base outline"
equation "d14 = length"
equation "d15 = width"
equation "d16 = baseoffset"
equation "d17 = baseoffset"
equation "d18 = thick"
equation "d20 = LtabWidth"
equation "d21 = LtabWidth"
equation "d22 = -thick"
equation "d24 = Ltab"
equation "d26 = length - LtabWidth * 3"
equation "d28 = -baseoffset"
equation "d29 = height"
equation "d30 = length"
equation "d31 = -thick"
equation "d33 = HtabWidth"
equation "d34 = HtabWidth"
equation "d35 = thick"
equation "d36 = -thick"
equation "d38 = Htab"
equation "d40 = height - HtabWidth * 3"
equation "d42 = -baseoffset"
equation "d43 = thick"
equation "d45 = thick"
equation "d46 = WtabWidth"
equation "d47 = WtabWidth"
equation "d48 = -thick"
equation "d50 = Wtab"
equation "d52 = width - WtabWidth * 3"
equation "d54 = -thick"
equation "d56 = -baseoffset - thick"
equation "d57 = thick"
equation "pot = 200 mm"
equation "d60 = pot"
equation "d62 = baseoffset * 2"
equation "d63 = -thick"
equation "spoutwidth = 30 mm"
equation "spoutcutdepth = 70 mm"
equation "d69 = spoutcutdepth"
equation "d70 = spoutwidth"
equation "d73 = spoutwidth"
equation "d74 = spoutcutdepth"
equation "d77 = spoutwidth"
equation "d78 = spoutcutdepth"
equation "d81 = WtabWidth"
equation "d82 = LtabWidth"
equation "d83 = thick"
equation "d84 = LtabWidth"
equation "d85 = LtabWidth"
equation "d86 = LtabWidth"
equation "d87 = LtabWidth"
equation "d88 = thick"
equation "d89 = WtabWidth"
equation "d90 = WtabWidth"
equation "d94 = WtabWidth"
equation "d106 = -thick"
equation "d108 = -thick"
equation "d110 = -thick"
equation "d112 = -thick"
equation "d114 = thick + 5 mm"
equation "d122 = -thick * 2"
equation "d124 = Ltab"
equation "d126 = length - LtabWidth * 3"
equation "d128 = thick + 5 mm"
equation "d129 = thick"
equation "d135 = -thick"
equation "d137 = -thick"
equation "d139 = -thick"
equation "d144 = thick"
equation "d156 = -thick"
equation "d159 = -thick"
equation "d162 = -thick"
equation "d194 = -thick"
equation "Sides = 69 mm"
equation "servolength = 22.75 mm"
equation "servowidth = 13 mm"
equation "thick_1 = 2 mm"
equation "spoutwidth_1 = 30 mm"
equation "servotab = 5 mm"
equation "spouthole = 15 mm"
equation "offset = 9 mm"
equation "slotlength = 24 mm"
equation "d199 = baseoffset"
equation "d200 = -thick"
